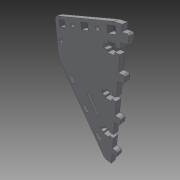
# Autodesk Inventor part: front_panel_brace_left
Saved by Autodesk Inventor 2014 (Build 180170000, 170)
## iProperties
Created: 2014-03-22
Part Number: front_panel_brace_left
Material: Plywood, Finish
Document SubType Name: Modeling
Designer: buben
Density: 0.552 g/cm^3
Appearance: Plywood - New
Author: buben
Autodesk Inventor part; units mm, degrees
ref_plane "YZ Plane" through (0, 0, 0) normal (1, 0, 0) x (0, 1, 0)
ref_plane "XZ Plane" through (0, 0, 0) normal (0, 1, 0) x (-1, 0, 0)
ref_plane "XY Plane" through (0, 0, 0) normal (0, 0, 1) x (1, 0, 0)
sketch "Sketch1" plane through (0, 0, 0) normal (0, 1, 0) x (-1, 0, 0)
  line L0 (8, 0) -> (76.1537, -12.0173)
  line L1 (76.1537, -12.0173) -> (76.1537, -54.5039)
  line L2 (76.1537, -54.5039) -> (9.2866, -150)
  line L3 (0, -150) -> (0, 0)
  line L4 (75.1537, -50.7018) -> (69.8292, -46.9735) construction
  line L5 (69.8292, -46.9735) -> (1, -145.2718) construction
  line L6 (1, -145.2718) -> (6.3245, -149) construction
  line L7 (6.3245, -149) -> (75.1537, -50.7018) construction
  line L8 (75.1537, -14.8873) -> (74.0249, -21.2885) construction
  line L9 (74.0249, -21.2885) -> (1, -8.4123) construction
  line L10 (1, -8.4123) -> (2.1287, -2.011) construction
  line L11 (2.1287, -2.011) -> (75.1537, -14.8873) construction
  line L12 (73.1537, -45.9735) -> (66.6537, -45.9735) construction
  line L13 (66.6537, -45.9735) -> (66.6537, -22.2885) construction
  line L14 (66.6537, -22.2885) -> (73.1537, -22.2885) construction
  line L15 (73.1537, -22.2885) -> (73.1537, -45.9735) construction
  line L16 (0, -150) -> (9.2866, -150)
  line L17 (0, 0) -> (8, 0)
  line L18 (66.6537, -51.5086) -> (66.6537, -19.9888)
  point P0 (0, 0)
  dimension "d0" = 6.5
  dimension "d1" = 3
  dimension "d2" = 3
  dimension "d3" = 3
  dimension "d4" = 120
  dimension "d5" = 80
  dimension "d6" = 35
  dimension "d7" = 1
  dimension "d8" = 1
  dimension "d9" = 1
  dimension "d10" = 1
  dimension "d12" = 1
  dimension "d13" = 8
  dimension "d14" = 150
  constraints: 38 end point, 8 parallel, 7 perpendicular, 2 equal length, 2 point on line, 2 vertical alignment, 1 coincident, 1 collinear, 1 horizontal, 1 vertical
  measures "d0" distance of L12.start L12.end
  measures "d1" distance between parallel lines of L2 L7
  measures "d2" distance between parallel lines of L1 L15
  measures "d3" distance between parallel lines of L0 L11
  measures "d4" distance of L4.end L5.end
  measures "d5" angle of L3 L0
  measures "d6" angle of L3 L2
  measures "d7" distance from line of L9.end L3
  measures "d8" distance from line of L8.start L1
  measures "d9" distance from line of L4.end L12
  measures "d10" distance from line of L8.end L14
  measures "d12" distance from line of L6.end L16
  measures "d13" distance of L3.end L0.start
  measures "d14" distance of L3.start L3.end
extrude "Extrusion1" add sketch "Sketch1" along normal blind 6.5
chamfer "Chamfer1" distance 2 angle 45 3 edges at (-76.1537, 3.25, -54.5039) (-76.1537, 3.25, -12.0173) (-9.2866, 3.25, -150)
sketch "Sketch3" plane through (0, 6.5, 0) normal (0, 1, 0) x (1, 0, 0)
  line L0 (-10.4338, 148.3617) -> (-75.0065, 56.1423) projected
  line L1 (-76.1537, 52.5039) -> (-76.1537, 14.0173) projected
  line L2 (-74.184, 11.67) -> (-8, 0) projected
  line L3 (0, 0) -> (0, 150) projected
  line L4 (0, 150) -> (-7.2866, 150) projected
  line L5 (-6.3245, 149) -> (-1, 145.2718) construction
  line L6 (-1, 145.2718) -> (-69.8292, 46.9735) construction
  line L7 (-69.8292, 46.9735) -> (-75.1537, 50.7018) construction
  line L8 (-75.1537, 50.7018) -> (-6.3245, 149) construction
  line L9 (-73.1537, 45.9735) -> (-66.6537, 45.9735) construction
  line L10 (-66.6537, 45.9735) -> (-66.6537, 22.2885) construction
  line L11 (-66.6537, 22.2885) -> (-73.1537, 22.2885) construction
  line L12 (-73.1537, 22.2885) -> (-73.1537, 45.9735) construction
  line L13 (-74.0249, 21.2885) -> (-75.1537, 14.8873) construction
  line L14 (-75.1537, 14.8873) -> (-2.1287, 2.011) construction
  line L15 (-2.1287, 2.011) -> (-1, 8.4123) construction
  line L16 (-1, 8.4123) -> (-74.0249, 21.2885) construction
  circle A0 centre (-69.9037, 34.131) radius 2.25
  line L17 (-56.0633, 66.6332) -> (-51.4747, 73.1864)
  line L18 (-51.4747, 73.1864) -> (-56.7992, 76.9146)
  line L19 (-56.7992, 76.9146) -> (-61.3878, 70.3614)
  line L20 (-61.3878, 70.3614) -> (-56.0633, 66.6332)
  line L21 (-37.7089, 92.846) -> (-33.1203, 99.3992)
  line L22 (-33.1203, 99.3992) -> (-38.4448, 103.1275)
  line L23 (-38.4448, 103.1275) -> (-43.0334, 96.5743)
  line L24 (-43.0334, 96.5743) -> (-37.7089, 92.846)
  line L25 (-19.3544, 119.0589) -> (-14.7658, 125.6121)
  line L26 (-14.7658, 125.6121) -> (-20.0903, 129.3404)
  line L27 (-20.0903, 129.3404) -> (-24.6789, 122.7871)
  line L28 (-24.6789, 122.7871) -> (-19.3544, 119.0589)
  line L29 (-72.4914, 48.8376) -> (-58.7256, 68.4973) construction
  line L30 (-54.137, 75.0505) -> (-40.3711, 94.7101) construction
  line L31 (-35.7825, 101.2634) -> (-22.0167, 120.923) construction
  line L32 (-17.4281, 127.4762) -> (-3.6622, 147.1359) construction
  line L33 (-16.3, 112.5) -> (-16.3, 108)
  line L34 (0, 108) -> (0, 112.5)
  line L35 (-12.3, 115) -> (-5, 115)
  line L36 (-5, 105.5) -> (-12.3, 105.5)
  line L37 (0, 112.5) -> (-5, 112.5)
  line L38 (-12.3, 112.5) -> (-16.3, 112.5)
  line L39 (-16.3, 108) -> (-12.3, 108)
  line L40 (-5, 108) -> (0, 108)
  line L41 (-12.3, 105.5) -> (-12.3, 108)
  line L42 (-12.3, 112.5) -> (-12.3, 115)
  line L43 (-5, 115) -> (-5, 112.5)
  line L44 (-5, 108) -> (-5, 105.5)
  line L45 (-70.0857, 20.5939) -> (-62.2073, 19.2048)
  line L46 (-62.2073, 19.2048) -> (-63.336, 12.8035)
  line L47 (-63.336, 12.8035) -> (-71.2144, 14.1927)
  line L48 (-71.2144, 14.1927) -> (-70.0857, 20.5939)
  line L49 (-41.4517, 15.545) -> (-33.5732, 14.1558)
  line L50 (-33.5732, 14.1558) -> (-34.702, 7.7546)
  line L51 (-34.702, 7.7546) -> (-42.5804, 9.1437)
  line L52 (-42.5804, 9.1437) -> (-41.4517, 15.545)
  line L53 (-12.8177, 10.496) -> (-4.9392, 9.1069)
  line L54 (-4.9392, 9.1069) -> (-6.0679, 2.7056)
  line L55 (-6.0679, 2.7056) -> (-13.9464, 4.0948)
  line L56 (-13.9464, 4.0948) -> (-12.8177, 10.496)
  line L57 (-62.7716, 16.0041) -> (-42.0161, 12.3444) construction
  line L58 (-34.1376, 10.9552) -> (-13.382, 7.2954) construction
  circle A1 centre (-52.3938, 14.1742) radius 2.25
  circle A2 centre (-23.7598, 9.1253) radius 2.25
  line L59 (-16.3, 67.975) -> (-16.3, 63.475)
  line L60 (0, 63.475) -> (0, 67.975)
  line L61 (-12.3, 70.475) -> (-5, 70.475)
  line L62 (-5, 60.975) -> (-12.3, 60.975)
  line L63 (0, 67.975) -> (-5, 67.975)
  line L64 (-12.3, 67.975) -> (-16.3, 67.975)
  line L65 (-16.3, 63.475) -> (-12.3, 63.475)
  line L66 (-5, 63.475) -> (0, 63.475)
  line L67 (-12.3, 60.975) -> (-12.3, 63.475)
  line L68 (-12.3, 67.975) -> (-12.3, 70.475)
  line L69 (-5, 70.475) -> (-5, 67.975)
  line L70 (-5, 63.475) -> (-5, 60.975)
  line L71 (-16.3, 23.45) -> (-16.3, 18.95)
  line L72 (0, 18.95) -> (0, 23.45)
  line L73 (-12.3, 25.95) -> (-5, 25.95)
  line L74 (-5, 16.45) -> (-12.3, 16.45)
  line L75 (0, 23.45) -> (-5, 23.45)
  line L76 (-12.3, 23.45) -> (-16.3, 23.45)
  line L77 (-16.3, 18.95) -> (-12.3, 18.95)
  line L78 (-5, 18.95) -> (0, 18.95)
  line L79 (-12.3, 16.45) -> (-12.3, 18.95)
  line L80 (-12.3, 23.45) -> (-12.3, 25.95)
  line L81 (-5, 25.95) -> (-5, 23.45)
  line L82 (-5, 18.95) -> (-5, 16.45)
  line L83 (-8.65, 105.5) -> (-8.65, 70.475) construction
  line L84 (-8.65, 60.975) -> (-8.65, 25.95) construction
  line L85 (-8, 0) -> (0, 0) projected
  point P0 (-69.9037, 45.9735)
  point P1 (-73.1537, 34.131)
  point P2 (-16.3, 21.2)
  dimension "d25" = 6.5
  dimension "d26" = 3
  dimension "d27" = 3
  dimension "d28" = 3
  dimension "d29" = 120
  dimension "d30" = 1
  dimension "d31" = 1
  dimension "d32" = 1
  dimension "d33" = 1
  dimension "d34" = 1
  dimension "d35" = 4.5
  dimension "d36" = 8
  dimension "d37" = 4.5
  dimension "d38" = 5
  dimension "d39" = 4
  dimension "d40" = 7.3
  dimension "d41" = 2.5
  dimension "d42" = 4
  dimension "d43" = 4
  dimension "d44" = 4.5
  dimension "d45" = 5
  dimension "d46" = 4
  dimension "d47" = 7.3
  dimension "d48" = 2.5
  dimension "d49" = 4.5
  dimension "d50" = 5
  dimension "d51" = 4
  dimension "d52" = 7.3
  dimension "d53" = 2.5
  dimension "d55" = 35
  dimension "d67" = 21.2
  constraints: 160 end point, 51 parallel, 27 collinear, 25 perpendicular, 21 midpoint, 16 equal length, 9 horizontal, 3 centre point, 2 equal radius, 1 horizontal alignment, 1 point on line, 1 vertical alignment
  measures "d25" distance of L5.start L5.end
  measures "d26" distance between parallel lines of L1 L12
  measures "d27" distance between parallel lines of L0 L8
  measures "d28" distance between parallel lines of L2 L14
  measures "d29" distance of L5.end L6.end
  measures "d30" distance from line of L4 L5.start
  measures "d31" distance from line of L6.end L9
  measures "d32" distance from line of L1 L13.end
  measures "d33" distance from line of L3 L15.end
  measures "d34" vertical distance of L13.start L11.end
  measures "d35" diameter of A0
  measures "d36" distance of L17.start L17.end
  measures "d37" distance of L33.start L33.end
  measures "d38" distance of L40.start L34.start
  measures "d39" distance of L33.end L39.end
  measures "d40" distance of L36.start L36.end
  measures "d41" distance of L36.end L39.end
  measures "d42" distance between parallel lines of L13 L48
  measures "d43" distance between parallel lines of L15 L54
  measures "d44" distance of L59.start L59.end
  measures "d45" distance of L70.start L60.start
  measures "d46" distance of L59.end L65.end
  measures "d47" distance of L62.start L67.start
  measures "d48" distance of L67.start L65.end
  measures "d49" distance of L71.start L71.end
  measures "d50" distance of L82.start L72.start
  measures "d51" distance of L71.end L77.end
  measures "d52" distance of L74.start L79.start
  measures "d53" distance of L79.start L77.end
  measures "d55" distance from line of L4 L35.start
  measures "d67" distance from line of L85 point (-16.3, 21.2)
extrude "Extrusion3" cut sketch "Sketch3" against normal through all
sketch "Sketch4" plane through (0, 6.5, 0) normal (0, 1, 0) x (1, 0, 0)
  line L0 (0, 67.975) -> (0, 108) projected
  line L1 (0, 112.5) -> (0, 150) projected
  line L2 (0, 0) -> (0, 18.95) projected
  line L3 (-16.3, 18.95) -> (-16.3, 23.45) projected
  line L4 (0, 23.45) -> (0, 63.475) projected
  line L5 (0, 135.25) -> (4.5, 135.25)
  line L6 (6.5, 133.25) -> (6.5, 129.25)
  line L7 (4.5, 127.25) -> (0, 127.25)
  line L8 (0, 127.25) -> (0, 135.25)
  line L9 (0, 91.9875) -> (4.5, 91.9875)
  line L10 (6.5, 89.9875) -> (6.5, 85.9875)
  line L11 (4.5, 83.9875) -> (0, 83.9875)
  line L12 (0, 83.9875) -> (0, 91.9875)
  line L13 (0, 47.4625) -> (4.5, 47.4625)
  line L14 (6.5, 45.4625) -> (6.5, 41.4625)
  line L15 (4.5, 39.4625) -> (0, 39.4625)
  line L16 (0, 39.4625) -> (0, 47.4625)
  line L17 (0, 13.7) -> (4.5, 13.7)
  line L18 (6.5, 11.7) -> (6.5, 7.7)
  line L19 (4.5, 5.7) -> (0, 5.7)
  line L20 (0, 5.7) -> (0, 13.7)
  arc A0 (6.5, 133.25) -> (4.5, 135.25) centre (4.5, 133.25) ccw
  arc A1 (4.5, 127.25) -> (6.5, 129.25) centre (4.5, 129.25) ccw
  arc A2 (6.5, 89.9875) -> (4.5, 91.9875) centre (4.5, 89.9875) ccw
  arc A3 (4.5, 83.9875) -> (6.5, 85.9875) centre (4.5, 85.9875) ccw
  arc A4 (6.5, 45.4625) -> (4.5, 47.4625) centre (4.5, 45.4625) ccw
  arc A5 (4.5, 39.4625) -> (6.5, 41.4625) centre (4.5, 41.4625) ccw
  arc A6 (6.5, 11.7) -> (4.5, 13.7) centre (4.5, 11.7) ccw
  arc A7 (4.5, 5.7) -> (6.5, 7.7) centre (4.5, 7.7) ccw
  point P0 (-16.3, 21.2)
  point P1 (6.5, 131.25)
  point P2 (0, 131.25)
  point P3 (6.5, 87.9875)
  point P4 (0, 87.9875)
  point P5 (6.5, 43.4625)
  point P6 (0, 43.4625)
  dimension "d58" = 2
  dimension "d59" = 8
  dimension "d60" = 8
  dimension "d61" = 8
  dimension "d62" = 8
  dimension "d63" = 6.5
  dimension "d64" = 7.5
  constraints: 32 end point, 16 point on circle, 16 tangent, 8 centre point, 8 parallel, 7 equal radius, 7 midpoint, 4 horizontal, 4 perpendicular, 4 point on line, 3 collinear, 3 horizontal alignment
  measures "d58" radius of A0
  measures "d59" distance between parallel lines of L7 L5
  measures "d60" distance between parallel lines of L11 L9
  measures "d61" distance between parallel lines of L15 L13
  measures "d62" distance between parallel lines of L19 L17
  measures "d63" distance between parallel lines of L1 L6
  measures "d64" distance from line of L17 point (-16.3, 21.2)
extrude "Extrusion4" add sketch "Sketch4" against normal blind 6.5
sketch "Sketch5" plane through (0, 6.5, 0) normal (0, 1, 0) x (1, 0, 0)
  line L0 (0, 150) -> (-7.2866, 150) projected
  line L1 (-10.4338, 148.3617) -> (-75.0065, 56.1423) projected
  line L2 (-20.9484, 97.6045) -> (-19.2282, 96.4) construction
  line L3 (-19.2282, 96.4) -> (-32.9941, 76.7404) construction
  line L4 (-32.9941, 76.7404) -> (-34.7143, 77.9449) construction
  line L5 (-34.7143, 77.9449) -> (-20.9484, 97.6045) construction
  line L6 (-32.8222, 75.7654) -> (-18.2533, 96.5719)
  line L7 (-18.2533, 96.5719) -> (-21.1203, 98.5794)
  line L8 (-21.1203, 98.5794) -> (-35.6892, 77.773)
  line L9 (-35.6892, 77.773) -> (-32.8222, 75.7654)
  dimension "d68" = 20.5
  dimension "d69" = 24
  dimension "d70" = 2.1
  dimension "d71" = 53.6
  dimension "d72" = 0.7
  constraints: 16 end point, 5 parallel, 2 perpendicular, 3 other
  measures "d68" distance between parallel lines of L1 L5
  measures "d69" distance of L4.end L2.start
  measures "d70" distance of L3.end L4.end
  measures "d71" distance from line of L2.end L0
  measures "d72" distance between parallel lines of L3 L6
extrude "Extrusion5" cut sketch "Sketch5" against normal through all
fillet "Fillet1" radius 0.3 4 edges at (-32.8222, 3.25, -75.7654) (-18.2533, 3.25, -96.5719) (-21.1203, 3.25, -98.5794) (-35.6892, 3.25, -77.773)
equation "\"d60\" = d59"
equation "\"d61\" = d60"
equation "\"d62\" = d61"
body "Solid1"
